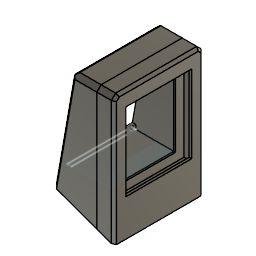
AIO-AIR-CASE-V2 (Autodesk Fusion 360 design; units mm, degrees)
Autodesk Fusion 360 part; units mm, degrees
note: some values were not read from the file. Chosen so that the rebuilt part matches the saved one: the sign of a taper; which pieces of a blend or face edit are solid.
sketch "Sketch1" plane through (0, 0, 0) normal (0, 1, 0) x (1, 0, 0)
sketch "Sketch2" plane through (0, 0, 0) normal (0, 0, 1) x (1, 0, 0)
sketch "Sketch3" plane through (0, 0, 0) normal (1, 0, 0) x (0, 1, 0)
  line L0 (0, 0) -> (-95, 0)
  line L1 (-95, 0) -> (-95, 115)
  line L2 (-95, 115) -> (0, 115)
  line L3 (0, 115) -> (0, 0)
  dimension "d1" = 95
  dimension "d2" = 115
  constraint horizontal L0
  constraint vertical L1
  constraint horizontal L2
  constraint vertical L3
  constraint coincident L0.start L3.end
  measures "d1" distance of L0.start L0.end
  measures "d2" distance of L0.start L2.end
other "Base Mesh Feature2"
other "Modify1"
extrude "Extrude1" add sketch "Sketch3" against normal blind 2 makes body 1
sketch "Sketch4" plane through (0, 0, 0) normal (1, 0, 0) x (0, 1, 0)
  line L0 (0, 115) -> (-95, 115)
  line L1 (-95, 115) -> (-95, 0)
  line L2 (-95, 0) -> (0, 0)
  line L3 (0, 0) -> (0, 115)
  line L4 (0, 115) -> (-95, 115)
  line L5 (-95, 115) -> (-95, 120)
  line L6 (-95, 120) -> (0, 120)
  line L7 (0, 120) -> (0, 115)
  line L8 (-95, 120) -> (-100, 120)
  line L9 (-100, 120) -> (-100, 0)
  line L10 (-100, 0) -> (-95, 0)
  line L11 (-95, 0) -> (-95, 120)
  line L12 (-100, 0) -> (0, 0)
  line L13 (0, 0) -> (0, -5)
  line L14 (0, -5) -> (-100, -5)
  line L15 (-100, -5) -> (-100, 0)
  line L16 (0, 120) -> (5, 120)
  line L17 (5, 120) -> (5, -5)
  line L18 (5, -5) -> (0, -5)
  line L19 (0, -5) -> (0, 120)
  constraint horizontal L4
  constraint vertical L5
  constraint horizontal L6
  constraint vertical L7
  constraint coincident L0.start L3.end
  constraint horizontal L8
  constraint vertical L9
  constraint horizontal L10
  constraint vertical L11
  constraint horizontal L12
  constraint vertical L13
  constraint horizontal L14
  constraint vertical L15
  constraint horizontal L16
  constraint vertical L17
  constraint horizontal L18
  constraint vertical L19
extrude "Extrude2" add sketch "Sketch4" along normal blind 15 separate body contours L3 L7 L13 L16 L17 L18 L19 | L0 L4 L5 L6 L7 L11 L19 | L1 L5 L8 L9 L10 L11 L12 | L2 L10 L12 L13 L14 L15 L19 makes body 2
sketch "Sketch5" plane through (15, 0, 0) normal (1, 0, 0) x (0, 1, 0)
  line L0 (0, 0) -> (-95, 0)
  line L1 (-95, 0) -> (-95, 115)
  line L2 (-95, 115) -> (0, 115)
  line L3 (0, 115) -> (0, 0)
  line L4 (5, 120) -> (-100, 120)
  line L5 (-100, 120) -> (-100, -5)
  line L6 (-100, -5) -> (5, -5)
  line L7 (5, -5) -> (5, 120)
  line L8 (-100, 120) -> (5, -5)
  line L9 (5, 120) -> (-100, -5)
  line L10 (-9, 12) -> (-86, 12)
  line L11 (-86, 12) -> (-86, 103)
  line L12 (-86, 103) -> (-9, 103)
  line L13 (-9, 103) -> (-9, 12)
  line L14 (-9, 12) -> (-86, 103) construction
  line L15 (-86, 12) -> (-9, 103) construction
  point P0 (-47.5, 57.5)
  dimension "d7" = 77
  dimension "d8" = 91
  constraint coincident L4.end L5.start
  constraint coincident L6.end L7.start
  constraint coincident L4.start L7.end
  constraint coincident L5.end L6.start
  constraint horizontal L10
  constraint perpendicular L10 L11
  constraint parallel L10 L12
  constraint parallel L11 L13
  constraint coincident L14 P0
  constraint coincident L15 P0
  constraint midpoint L9 P0
  measures "d7" distance of L11.end L12.end
  measures "d8" distance of L10.end L11.end
extrude "Extrude3" add sketch "Sketch5" along normal blind 3 separate body contours L0 L1 L3 L6 L8 L9 | L0 L1 L3 L8 L9 L10 | L3 L8 L9 L10 L12 L13 | L3 L7 L8 L9 | L1 L5 L8 L9 | L1 L8 L9 L10 L11 L12 | L1 L2 L3 L8 L9 L12 | L1 L2 L3 L4 L8 L9 makes body 3
sketch "Sketch6" plane through (-2, 0, 0) normal (-1, 0, 0) x (0, -1, 0)
  line L0 (95, 115) -> (0, 115)
  line L1 (0, 115) -> (0, 0)
  line L2 (0, 0) -> (95, 0)
  line L3 (95, 0) -> (95, 115)
  circle A0 centre (3.1, 111.25) radius 1.1
  circle A1 centre (92, 111.25) radius 1.1
  circle A2 centre (91.9973, 2.254) radius 1.104
extrude "Extrude4" cut sketch "Sketch6" against normal blind 5 contours A0 | A1 | A2 bodies 1
sketch "Sketch7" plane through (-2, 0, 0) normal (-1, 0, 0) x (0, -1, 0)
  circle A0 centre (3.1, 111.25) radius 1.1
  circle A1 centre (92, 111.25) radius 1.1
  circle A2 centre (91.9973, 2.254) radius 1.104
  line L0 (95, 115) -> (0, 115)
  line L1 (0, 115) -> (0, 0)
  line L2 (0, 0) -> (95, 0)
  line L3 (95, 0) -> (95, 115)
  line L4 (10, 105) -> (85, 105)
  line L5 (85, 105) -> (85, 10)
  line L6 (85, 10) -> (10, 10)
  line L7 (10, 10) -> (10, 105)
  constraint horizontal L4
  constraint vertical L5
  constraint horizontal L6
  constraint vertical L7
extrude "Extrude5" cut sketch "Sketch7" against normal blind 5 contours L4 L5 L6 L7 bodies 1
extrude "Extrude6" add 1 faces at (-0.6667, -63.3333, 115) along direction (0, 0, 1) blind 5 on bodies 1 bodies 1 3 2
extrude "Extrude7" add 1 faces at (-1.3333, -95, 78.3333) along direction (0, -1, 0) blind 5 on bodies 1 bodies 1
extrude "Extrude8" add 1 faces at (-1.3333, -65, 0) along direction (0, 0, -1) blind 5 on bodies 1 bodies 1
extrude "Extrude9" add 1 faces at (-1.3333, 0, 76.6667) along direction (0, 1, 0) blind 5 on bodies 1 bodies 1
sketch "Sketch8" plane through (-2, 0, 0) normal (-1, 0, 0) x (0, -1, 0)
  line L0 (85, 105) -> (85, 10)
  line L1 (85, 10) -> (10, 10)
  line L2 (10, 10) -> (10, 105)
  line L3 (10, 105) -> (85, 105)
  circle A0 centre (3.1, 111.25) radius 1.1
  circle A1 centre (92, 111.25) radius 1.1
  circle A2 centre (91.9973, 2.254) radius 1.104
  line L4 (-5, -5) -> (100, -5)
  line L5 (100, -5) -> (100, 120)
  line L6 (100, 120) -> (-5, 120)
  line L7 (-5, 120) -> (-5, -5)
  line L8 (-5, 120) -> (100, 120)
  line L9 (100, 120) -> (100, -5)
  line L10 (100, -5) -> (-5, -5)
  line L11 (-5, -5) -> (-5, 120)
  constraint horizontal L8
  constraint vertical L9
  constraint horizontal L10
  constraint vertical L11
  constraint coincident L4.end L5.start
  constraint coincident L6.end L7.start
extrude "Extrude10" add sketch "Sketch8" along normal blind 30 separate body makes body 4
draft "Draft1" angle -10 neutral plane through (-2, -100, 120) pull (0, 0, -1) 1 faces at (-32, -2.4599, 38.4729) on bodies 4
draft "Draft2" angle 20 neutral plane through (-52.8378, 0, 1.8231) pull (-0.984808, 0, 0.173648) 3 faces at (16, -65, -5) (9.3333, -65, -5) (-19.347, -30, -5) on bodies 1 3 4
chamfer "Chamfer1" distance 5 angle 45 6 edges at (6.5, 5, 120) (6.5, -100, 120) (16.5, 5, 120) (16.5, -100, 120) (-17, 5, 120) (-17, -100, 120) on bodies 1 3 4
chamfer "Chamfer2" distance 5 angle 45 1 edges at (-32, -47.5, 120) on bodies 4
chamfer "Chamfer3" distance 3 angle 45 5 edges at (18, -47.5, 120) (18, -97.5, 117.5) (18, -100, 41.8896) (18, 5, 41.8896) (18, 2.5, 117.5) on bodies 3
chamfer "Chamfer4" distance 5 angle 45 2 edges at (-43.4613, -100, 55) (-43.4613, 5, 55) on bodies 4
sketch "Sketch9" plane through (0, 0, 10) normal (0, 0, 1) x (-1, 0, 0)
  line L0 (2, 85) -> (2, 10)
  line L1 (2, 10) -> (51.396, 10)
  line L2 (51.396, 10) -> (51.396, 85)
  line L3 (51.396, 85) -> (2, 85)
  line L4 (51.396, 10) -> (46.396, 10)
  line L5 (46.396, 10) -> (46.396, 85)
  line L6 (46.396, 85) -> (51.396, 85)
  line L7 (51.396, 85) -> (51.396, 10)
  line L8 (51.396, 10) -> (46.396, 10)
  dimension "d33" = 5
  constraint horizontal L4
  constraint vertical L5
  constraint horizontal L6
  constraint vertical L7
  constraint coincident L1.end L2.start
  measures "d33" distance of L1.end L4.end
sketch "Sketch10" plane through (0, -10, 0) normal (0, -1, 0) x (1, 0, 0)
  line L0 (-2, 10) -> (-2, 105)
  line L1 (-2, 105) -> (-34.6449, 105)
  line L2 (-34.6449, 105) -> (-51.396, 10)
  line L3 (-51.396, 10) -> (-2, 10)
  line L4 (-46.4, 10) -> (-51.396, 10)
  line L5 (-51.396, 10) -> (-50.5181, 14.9784)
  line L6 (-46.4, 10) -> (-46.4, 14.9784)
  line L7 (-46.4, 14.9784) -> (-50.5181, 14.9784)
  constraint coincident L3 L4.start
  constraint coincident L2.end L3.start
  constraint coincident L2 L5.end
  constraint perpendicular L3 L6
  constraint perpendicular L6 L7
extrude "Extrude11" add sketch "Sketch10" along normal blind 75 separate body contours L2 L3 L4 L5 L6 L7 makes body 5
sketch "Sketch11" plane through (-51.5563, 0, 9.0908) normal (-0.984808, 0, 0.173648) x (0, -1, 0)
  line L0 (10, 5.9785) -> (10, 0.9233)
  line L1 (10, 0.9233) -> (85, 0.9233)
  line L2 (85, 0.9233) -> (85, 5.9785)
  line L3 (85, 5.9785) -> (10, 5.9785)
  line L4 (10, 5.9785) -> (85, 0.9233)
  line L5 (85, 5.9785) -> (10, 0.9233)
  line L6 (51.75, 2.2009) -> (43.25, 2.2009)
  line L7 (43.25, 2.2009) -> (43.25, 4.7009)
  line L8 (43.25, 4.7009) -> (51.75, 4.7009)
  line L9 (51.75, 4.7009) -> (51.75, 2.2009)
  line L10 (51.75, 2.2009) -> (43.25, 4.7009) construction
  line L11 (43.25, 2.2009) -> (51.75, 4.7009) construction
  point P0 (47.5, 3.4509)
  dimension "d36" = 8.5
  dimension "d37" = 2.5
  constraint coincident L0.start L3.end
  constraint coincident L1.end L2.start
  constraint coincident L2.end L3.start
  constraint coincident L0.end L1.start
  constraint horizontal L6
  constraint perpendicular L6 L7
  constraint parallel L6 L8
  constraint parallel L7 L9
  constraint coincident L10 P0
  constraint coincident L11 P0
  constraint midpoint L4 P0
  measures "d36" distance of L7.end L8.end
  measures "d37" distance of L6.end L7.end
extrude "Extrude12" cut sketch "Sketch11" against normal blind 5 contours L4 L5 L7 L8 L9 | L4 L5 L7 | L4 L5 L6 L7 L9 | L4 L5 L9 bodies 5
fillet "Fillet1" radius 0.5 2 edges at (-48.7871, -51.75, 10.8373) (-48.57, -51.75, 13.3376) on bodies 5
fillet "Fillet2" radius 0.5 2 edges at (-48.7871, -43.25, 10.8373) (-48.57, -43.25, 13.3376) on bodies 5
